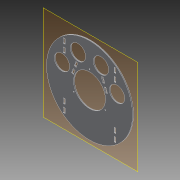
# Autodesk Inventor part: Основание емкости
Saved by Autodesk Inventor 2022 (Build 260153000, 153)
## iProperties
Created: 2025-01-25
Part Number: Основание емкости
Material: Типовые
Document SubType Name: Modeling
Designer: Ivan
Density: 1 g/cm^3
Appearance: По умолчанию
Author: Ivan
Autodesk Inventor part; units mm, degrees
ref_plane "YZ Plane" through (0, 0, 0) normal (1, 0, 0) x (0, 1, 0)
ref_plane "XZ Plane" through (0, 0, 0) normal (0, 1, 0) x (-1, 0, 0)
ref_plane "XY Plane" through (0, 0, 0) normal (0, 0, 1) x (1, 0, 0)
ref_plane "РабПлоскость1" through (0, 0, 3) normal (0, 0, 1) x (1, 0, 0)
sketch "Эскиз1" plane through (0, 0, 3) normal (0, 0, 1) x (1, 0, 0)
  circle A0 centre (0, 0) radius 50 projected
  circle A1 centre (0, 0) radius 135 projected
  line L0 (0, 0) -> (0, 161.4667) construction
  line L1 (0, 0) -> (-129.0077, -129.0077) construction
  line L2 (0, 0) -> (141.934, -141.934) construction
  line L3 (0, 0) -> (-189.6915, 0) construction
  line L4 (0, 0) -> (168.8407, 0) construction
  circle A2 centre (0, 0) radius 92.5 construction
  line L5 (0, 135) -> (0, 50) construction
  line L6 (0, 0) -> (-61.9345, 145.9085) construction
  line L7 (0, 0) -> (-163.7095, 62.8422) construction
  circle A3 centre (-36.1426, 85.1467) radius 26.5
  circle A4 centre (-86.3562, 33.149) radius 26.5
  circle A5 centre (36.1426, 85.1467) radius 26.5
  circle A6 centre (86.3562, 33.149) radius 26.5
  line L8 (-89.8562, 61.649) -> (-82.8562, 61.649) construction
  line L9 (-82.8562, 61.649) -> (-82.8562, 74.649) construction
  line L10 (-82.8562, 74.649) -> (-89.8562, 74.649) construction
  line L11 (-89.8562, 74.649) -> (-89.8562, 61.649) construction
  line L12 (-89.8562, 61.649) -> (-82.8562, 74.649) construction
  line L13 (-82.8562, 61.649) -> (-89.8562, 74.649) construction
  line L14 (-82.8562, 61.649) -> (-76.8562, 61.649)
  line L15 (-76.8562, 61.649) -> (-76.8562, 101.649)
  line L16 (-76.8562, 101.649) -> (-82.8562, 101.649)
  line L17 (-82.8562, 101.649) -> (-82.8562, 61.649)
  line L18 (-82.8562, 61.649) -> (-76.8562, 101.649) construction
  line L19 (-76.8562, 61.649) -> (-82.8562, 101.649) construction
  line L20 (-79.8562, 81.649) -> (-76.8562, 81.649) construction
  line L21 (-82.8562, 76.649) -> (-76.8562, 76.649)
  line L22 (-82.8562, 86.649) -> (-76.8562, 86.649)
  line L23 (82.8562, 61.649) -> (82.8562, 74.649) construction
  line L24 (82.8562, 61.649) -> (76.8562, 61.649)
  line L25 (76.8562, 61.649) -> (76.8562, 101.649)
  line L26 (76.8562, 101.649) -> (82.8562, 101.649)
  line L27 (82.8562, 101.649) -> (82.8562, 61.649)
  line L28 (82.8562, 61.649) -> (76.8562, 101.649) construction
  line L29 (76.8562, 61.649) -> (82.8562, 101.649) construction
  line L30 (79.8562, 81.649) -> (76.8562, 81.649) construction
  line L31 (82.8562, 76.649) -> (76.8562, 76.649)
  line L32 (82.8562, 86.649) -> (76.8562, 86.649)
  line L33 (-82.8562, -61.649) -> (-82.8562, -74.649) construction
  line L34 (-82.8562, -61.649) -> (-76.8562, -61.649)
  line L35 (-76.8562, -61.649) -> (-76.8562, -101.649)
  line L36 (-76.8562, -101.649) -> (-82.8562, -101.649)
  line L37 (-82.8562, -101.649) -> (-82.8562, -61.649)
  line L38 (-82.8562, -61.649) -> (-76.8562, -101.649) construction
  line L39 (-76.8562, -61.649) -> (-82.8562, -101.649) construction
  line L40 (-79.8562, -81.649) -> (-76.8562, -81.649) construction
  line L41 (-82.8562, -76.649) -> (-76.8562, -76.649)
  line L42 (-82.8562, -86.649) -> (-76.8562, -86.649)
  line L43 (82.8562, -61.649) -> (76.8562, -61.649)
  line L44 (79.8562, -81.649) -> (76.8562, -81.649) construction
  line L45 (82.8562, -86.649) -> (76.8562, -86.649)
  line L46 (82.8562, -101.649) -> (82.8562, -61.649)
  line L47 (82.8562, -61.649) -> (76.8562, -101.649) construction
  line L48 (76.8562, -61.649) -> (76.8562, -101.649)
  line L49 (76.8562, -61.649) -> (82.8562, -101.649) construction
  line L50 (76.8562, -101.649) -> (82.8562, -101.649)
  line L51 (82.8562, -76.649) -> (76.8562, -76.649)
  line L52 (82.8562, -61.649) -> (82.8562, -74.649) construction
  line L53 (-36.1426, 85.1467) -> (-62.0654, 13.9246) construction
  line L54 (-53.6254, 47.3465) -> (-49.1791, 59.5625) construction
  line L55 (-49.1791, 59.5625) -> (-42.6013, 57.1684) construction
  line L56 (-42.6013, 57.1684) -> (-47.0475, 44.9524) construction
  line L57 (-47.0475, 44.9524) -> (-53.6254, 47.3465) construction
  line L58 (-53.6254, 47.3465) -> (-42.6013, 57.1684) construction
  line L59 (-49.1791, 59.5625) -> (-47.0475, 44.9524) construction
  line L60 (-56.2821, 19.5807) -> (-42.6013, 57.1684)
  line L61 (-42.6013, 57.1684) -> (-36.9631, 55.1163)
  line L62 (-36.9631, 55.1163) -> (-50.6439, 17.5286)
  line L63 (-50.6439, 17.5286) -> (-56.2821, 19.5807)
  line L64 (-56.2821, 19.5807) -> (-36.9631, 55.1163) construction
  line L65 (-42.6013, 57.1684) -> (-50.6439, 17.5286) construction
  line L66 (-46.6226, 37.3485) -> (-43.8035, 36.3224) construction
  line L67 (-47.7316, 43.073) -> (-42.0934, 41.0209)
  line L68 (-51.1518, 33.6761) -> (-45.5136, 31.624)
  line L69 (53.6254, 47.3465) -> (49.1791, 59.5625) construction
  line L70 (49.1791, 59.5625) -> (42.6013, 57.1684) construction
  line L71 (42.6013, 57.1684) -> (47.0475, 44.9524) construction
  line L72 (47.0475, 44.9524) -> (53.6254, 47.3465) construction
  line L73 (53.6254, 47.3465) -> (42.6013, 57.1684) construction
  line L74 (49.1791, 59.5625) -> (47.0475, 44.9524) construction
  line L75 (56.2821, 19.5807) -> (42.6013, 57.1684)
  line L76 (42.6013, 57.1684) -> (36.9631, 55.1163)
  line L77 (36.9631, 55.1163) -> (50.6439, 17.5286)
  line L78 (50.6439, 17.5286) -> (56.2821, 19.5807)
  line L79 (56.2821, 19.5807) -> (36.9631, 55.1163) construction
  line L80 (42.6013, 57.1684) -> (50.6439, 17.5286) construction
  line L81 (46.6226, 37.3485) -> (43.8035, 36.3224) construction
  line L82 (47.7316, 43.073) -> (42.0934, 41.0209)
  line L83 (51.1518, 33.6761) -> (45.5136, 31.624)
  line L84 (-42.6013, 57.1684) -> (-36.9631, 55.1163) projected
  line L85 (-36.9631, 55.1163) -> (-42.0934, 41.0209) projected
  line L86 (-42.0934, 41.0209) -> (-47.7316, 43.073) projected
  line L87 (-47.7316, 43.073) -> (-42.6013, 57.1684) projected
  line L88 (82.8562, 61.649) -> (76.8562, 61.649) projected
  line L89 (76.8562, 61.649) -> (76.8562, 76.649) projected
  line L90 (76.8562, 76.649) -> (82.8562, 76.649) projected
  line L91 (82.8562, 76.649) -> (82.8562, 61.649) projected
  line L92 (-82.8562, -76.649) -> (-82.8562, -61.649) projected
  line L93 (-82.8562, -61.649) -> (-76.8562, -61.649) projected
  line L94 (-76.8562, -61.649) -> (-76.8562, -76.649) projected
  line L95 (-76.8562, -76.649) -> (-82.8562, -76.649) projected
  line L96 (82.8562, -86.649) -> (82.8562, -101.649) projected
  line L97 (82.8562, -101.649) -> (76.8562, -101.649) projected
  line L98 (76.8562, -101.649) -> (76.8562, -86.649) projected
  line L99 (76.8562, -86.649) -> (82.8562, -86.649) projected
  line L100 (51.1518, 33.6761) -> (56.2821, 19.5807) projected
  line L101 (56.2821, 19.5807) -> (50.6439, 17.5286) projected
  line L102 (50.6439, 17.5286) -> (45.5136, 31.624) projected
  line L103 (45.5136, 31.624) -> (51.1518, 33.6761) projected
  line L104 (-76.8562, 61.649) -> (-82.8562, 61.649) projected
  line L105 (-82.8562, 61.649) -> (-82.8562, 76.649) projected
  line L106 (-82.8562, 76.649) -> (-76.8562, 76.649) projected
  line L107 (-76.8562, 76.649) -> (-76.8562, 61.649) projected
  line L108 (-45.5136, 31.624) -> (-50.6439, 17.5286) projected
  line L109 (-50.6439, 17.5286) -> (-56.2821, 19.5807) projected
  line L110 (-56.2821, 19.5807) -> (-51.1518, 33.6761) projected
  line L111 (-51.1518, 33.6761) -> (-45.5136, 31.624) projected
  line L112 (76.8562, 86.649) -> (76.8562, 101.649) projected
  line L113 (76.8562, 101.649) -> (82.8562, 101.649) projected
  line L114 (82.8562, 101.649) -> (82.8562, 86.649) projected
  line L115 (82.8562, 86.649) -> (76.8562, 86.649) projected
  line L116 (-76.8562, -101.649) -> (-82.8562, -101.649) projected
  line L117 (-82.8562, -101.649) -> (-82.8562, -86.649) projected
  line L118 (-82.8562, -86.649) -> (-76.8562, -86.649) projected
  line L119 (-76.8562, -86.649) -> (-76.8562, -101.649) projected
  line L120 (76.8562, -61.649) -> (82.8562, -61.649) projected
  line L121 (82.8562, -61.649) -> (82.8562, -76.649) projected
  line L122 (82.8562, -76.649) -> (76.8562, -76.649) projected
  line L123 (76.8562, -76.649) -> (76.8562, -61.649) projected
  line L124 (36.9631, 55.1163) -> (42.6013, 57.1684) projected
  line L125 (42.6013, 57.1684) -> (47.7316, 43.073) projected
  line L126 (47.7316, 43.073) -> (42.0934, 41.0209) projected
  line L127 (42.0934, 41.0209) -> (36.9631, 55.1163) projected
  line L128 (-82.8562, 86.649) -> (-82.8562, 101.649) projected
  line L129 (-82.8562, 101.649) -> (-76.8562, 101.649) projected
  line L130 (-76.8562, 101.649) -> (-76.8562, 86.649) projected
  line L131 (-76.8562, 86.649) -> (-82.8562, 86.649) projected
  circle A7 centre (49.7965, -28.75) radius 1.6 projected
  circle A8 centre (-49.7965, -28.75) radius 1.6 projected
  circle A9 centre (0, 57.5) radius 1.6 projected
  point P0 (0, 92.5)
  point P1 (-86.3562, 68.149)
  point P2 (-86.3562, 68.149)
  point P3 (-86.3562, -68.149)
  point P4 (-86.3562, -68.149)
  point P5 (-48.1133, 52.2575)
  point P6 (62.0654, 13.9246)
  point P7 (48.1133, 52.2575)
  dimension "d0" = 90
  dimension "d2" = 53
  dimension "d3" = 46
  dimension "d4" = 23
  dimension "d5" = 13
  dimension "d6" = 7
  dimension "d7" = 35
  dimension "d8" = 40
  dimension "d9" = 6
  dimension "d10" = 15
  dimension "d12" = 35
  dimension "d13" = 15
  dimension "d14" = 20
  constraints: 168 end point, 56 symmetric about line, 29 point on line, 22 midpoint, 9 parallel, 7 perpendicular, 5 centre point, 5 horizontal, 4 collinear, 4 equal length, 3 point on circle, 3 vertical alignment, 1 coincident, 1 equal radius, 1 vertical, 7 other
  measures "d0" angle of L2 L1
  measures "d2" diameter of A3
  measures "d3" angle of L7 L6
  measures "d4" angle of L0 L6
  measures "d5" distance of L10.end L8.start
  measures "d6" distance of L9.end L10.end
  measures "d7" distance of A4.centre point (-86.356, 68.149)
  measures "d8" distance of L14.end L15.end
  measures "d9" distance of L15.end L16.end
  measures "d10" distance between parallel lines of L22 L16
  measures "d12" distance of point (-48.113, 52.257) L53.start
  measures "d13" distance between parallel lines of L61 L67
  measures "d14" angle of L0 L53
extrude "Выдавливание1" add sketch "Эскиз1" along normal blind 3 contours A1 | L17 L22 L15 L21 | L31 L25 L32 L27 | L41 L35 L42 L37 | L46 L45 L48 L51 | L60 L67 L62 L68 | L83 L77 L82 L75 | A7 | A8 | A9
sketch "Эскиз2" plane through (0, 0, 6) normal (0, 0, 1) x (1, 0, 0)
  circle A0 centre (0, 0) radius 57.5 construction
  line L0 (0, 0) -> (0, 68.3153) construction
  point P0 (0, 0)
  point P1 (0, 57.5)
  dimension "d17" = 115
  constraints: 2 end point, 1 coincident, 1 point on line, 1 vertical, 1 vertical alignment, 2 other
hole "Отверстие1" at (0, 57.5, 6) direction (0, 0, -1) diameter 3.2 end through all clearance for "болты с шестигранной головкой / гайка ГОСТ 12876-67" size "M3" standard "ГОСТ"
pattern_circular "Круговой массив1" count 3 over 360 about axis through (0, 0, 3) along (0, 0, 1) of "Отверстие1"
sketch "Эскиз3" plane through (0, 0, 6) normal (0, 0, 1) x (1, 0, 0)
  circle A0 centre (86.3562, 33.149) radius 26.5
  circle A1 centre (36.1426, 85.1467) radius 26.5
  circle A2 centre (-36.1426, 85.1467) radius 26.5
  circle A3 centre (-86.3562, 33.149) radius 26.5
  circle A4 centre (86.3562, 33.149) radius 24
  circle A5 centre (36.1426, 85.1467) radius 24
  circle A6 centre (-36.1426, 85.1467) radius 24
  circle A7 centre (-86.3562, 33.149) radius 24
  point P0 (0, 0)
  dimension "d28" = 48
  constraints: 8 centre point, 4 coincident, 3 equal radius
  measures "d28" diameter of A4
extrude "Выдавливание2" add sketch "Эскиз3" against normal blind 3
equation "\"d4\" = 0.5 * d3"
equation "\"d12\" = d7"
equation "\"d13\" = d10"
